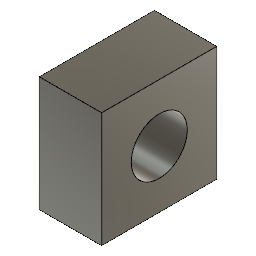
ANTEBRAZO COMPLETO v7 (Autodesk Fusion 360 archive; units mm, degrees)
design "UNION CON HUECO PARA CILINDR"
Autodesk Fusion 360 part; units mm, degrees
sketch "Boceto1" plane through (0, 0, 0) normal (1, 0, 0) x (0, 1, 0)
  line L0 (0, 0) -> (0, 35)
  line L1 (0, 35) -> (35, 35)
  line L2 (35, 35) -> (35, 0)
  line L3 (35, 0) -> (0, 0)
  dimension "d1" = 35
  dimension "d2" = 35
  constraint coincident L0.start L3.end
  constraint vertical L0
  constraint perpendicular L0 L1
  constraint perpendicular L1 L2
  constraint perpendicular L0 L3
  measures "d1" distance of L0.start L0.end
  measures "d2" distance of L0.end L1.end
extrude "Extruir1" add sketch "Boceto1" along normal blind 19
sketch "Boceto2" plane through (19, 0, 0) normal (1, 0, 0) x (0, 1, 0)
  line L0 (35, 0) -> (35, 35)
  line L1 (35, 35) -> (0, 35)
  line L2 (0, 35) -> (0, 0)
  line L3 (0, 0) -> (35, 0)
  circle A0 centre (17.5, 17.5) radius 8.5
  dimension "d5" = 17
  measures "d5" diameter of A0
extrude "Extruir2" cut sketch "Boceto2" against normal blind 15 contours A0

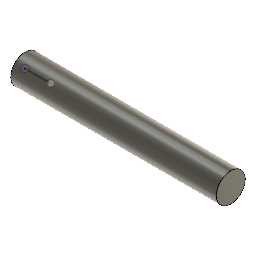
design "CILINDRO ANTEBRAZO"
Autodesk Fusion 360 part; units mm, degrees
cylinder "CilindroPrimitivo1" add diameter 17 height 200 placed x (0, 0, -1) y (0, 1, 0) z (1, 0, 0) at (0, 0, 0)
sketch "Boceto2" plane through (0, 0, 0) normal (0, 1, 0) x (1, 0, 0)
  line L0 (0, 0) -> (15, 0)
  constraint coincident L0.start origin
  constraint horizontal L0
extrude "Extruir1" cut 1 faces at (200, 1.6235, -2.7075) along direction (-1, 0, 0) blind 20
extrude "Extruir2" cut 1 faces at (180, 1.6235, -2.7075) along direction (-1, 0, 0) blind 30
extrude "Extruir3" cut 1 faces at (150, 1.6235, -2.7075) along direction (-1, 0, 0) blind 30
